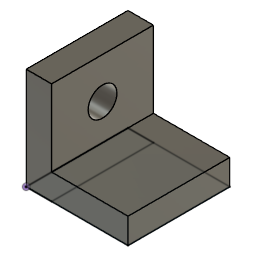
Final build (Autodesk Fusion 360 archive; units mm, degrees)
design "90 degree mount for coil housing"
part number: 2026-08-06-22-44-02-065
Autodesk Fusion 360 part; units mm, degrees
sketch "Sketch1" plane through (0, 0, 0) normal (0, 0, 1) x (1, 0, 0)
  line L0 (0, 0) -> (25.4, 0)
  line L1 (25.4, 0) -> (25.4, 25.4)
  line L2 (25.4, 25.4) -> (0, 25.4)
  line L3 (0, 25.4) -> (0, 0)
  line L4 (0, 25.4) -> (6.35, 25.4)
  line L5 (6.35, 25.4) -> (6.35, 0)
  line L6 (6.35, 0) -> (0, 0)
  line L7 (0, 0) -> (0, 25.4)
  dimension "d1" = 25.4
  dimension "d2" = 25.4
  dimension "d3" = 6.35
  constraint horizontal L0
  constraint vertical L1
  constraint horizontal L2
  constraint vertical L3
  constraint coincident L0.start L3.end
  constraint horizontal L4
  constraint vertical L5
  constraint horizontal L6
  constraint vertical L7
  constraint coincident L0 L5.end
  measures "d1" distance of L0.start L0.end
  measures "d2" distance of L0.start L2.end
  measures "d3" distance of L2.end L4.end
extrude "Extrude1" add sketch "Sketch1" along normal blind 6.35 contours L0 L1 L2 L5
extrude "Extrude2" add sketch "Sketch1" along normal blind 25.4 contours L0 L2 L3 L4 L5 L6 L7
sketch "Sketch2" plane through (6.35, 0, 0) normal (1, 0, 0) x (0, 1, 0)
  line L0 (0, 6.35) -> (25.4, 6.35)
  line L1 (25.4, 6.35) -> (25.4, 25.4)
  line L2 (25.4, 25.4) -> (0, 25.4)
  line L3 (0, 25.4) -> (0, 6.35)
  circle A0 centre (12.7, 15.24) radius 3.5921
extrude "Extrude3" cut sketch "Sketch2" against normal blind 38.1 contours A0

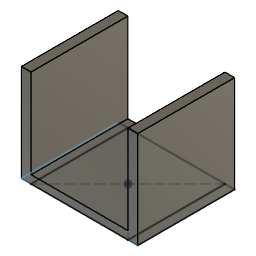
design "arm holder"
part number: 2026-08-05-14-50-43-195
Autodesk Fusion 360 part; units mm, degrees
sketch "Sketch1" plane through (0, 0, 0) normal (0, 0, 1) x (1, 0, 0)
  line L0 (38.1, 38.1) -> (-38.1, 38.1)
  line L1 (-38.1, 38.1) -> (-38.1, -38.1)
  line L2 (-38.1, -38.1) -> (38.1, -38.1)
  line L3 (38.1, -38.1) -> (38.1, 38.1)
  line L4 (38.1, 38.1) -> (-38.1, -38.1) construction
  line L5 (-38.1, 38.1) -> (38.1, -38.1) construction
  line L6 (-38.1, 38.1) -> (-45.72, 38.1)
  line L7 (-45.72, 38.1) -> (-45.72, -38.1)
  line L8 (-45.72, -38.1) -> (-38.1, -38.1)
  line L9 (-38.1, -38.1) -> (-38.1, 38.1)
  line L10 (38.1, 38.1) -> (45.72, 38.1)
  line L11 (45.72, 38.1) -> (45.72, -38.1)
  line L12 (45.72, -38.1) -> (38.1, -38.1)
  line L13 (38.1, -38.1) -> (38.1, 38.1)
  dimension "d1" = 76.2
  dimension "d2" = 76.2
  dimension "d3" = 7.62
  constraint horizontal L0
  constraint perpendicular L0 L1
  constraint parallel L0 L2
  constraint parallel L1 L3
  constraint coincident L4 origin
  constraint coincident L5 origin
  constraint horizontal L6
  constraint vertical L7
  constraint horizontal L8
  constraint vertical L9
  constraint horizontal L10
  constraint vertical L11
  constraint horizontal L12
  constraint vertical L13
  measures "d1" distance of L1.end L2.end
  measures "d2" distance of L0.end L1.end
  measures "d3" distance of L0.start L10.end
extrude "Extrude1" add sketch "Sketch1" along normal blind 6.35 contours L0 L1 L2 L3 L9 L13
sketch "Sketch2" plane through (0, 0, 0) normal (0, 0, 1) x (1, 0, 0)
extrude "Extrude2" add sketch "Sketch1" along normal blind 76.2 contours L3 L10 L11 L12 L13 | L1 L6 L7 L8 L9

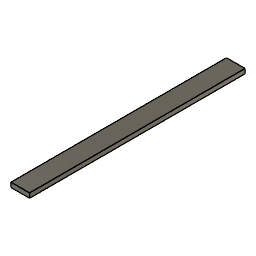
design "front and back side plates for coil housing"
part number: 2026-08-05-15-19-59-138
Autodesk Fusion 360 part; units mm, degrees
sketch "Sketch1" plane through (0, 0, 0) normal (0, 0, 1) x (1, 0, 0)
  line L0 (0, 0) -> (25.4, 0)
  line L1 (25.4, 0) -> (25.4, 293.37)
  line L2 (25.4, 293.37) -> (0, 293.37)
  line L3 (0, 293.37) -> (0, 0)
  dimension "d1" = 25.4
  dimension "d2" = 293.37
  constraint horizontal L0
  constraint vertical L1
  constraint horizontal L2
  constraint vertical L3
  constraint coincident L0.start L3.end
  measures "d1" distance of L0.start L0.end
  measures "d2" distance of L0.start L2.end
extrude "Extrude1" add sketch "Sketch1" along normal blind 6.35

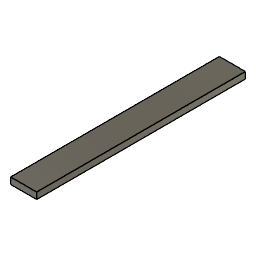
design "coil housing side plates"
part number: 2026-08-05-15-19-17-002
Autodesk Fusion 360 part; units mm, degrees
sketch "Sketch1" plane through (0, 0, 0) normal (0, 0, 1) x (1, 0, 0)
  line L0 (0, 0) -> (25.4, 0)
  line L1 (25.4, 0) -> (25.4, 203.2)
  line L2 (25.4, 203.2) -> (0, 203.2)
  line L3 (0, 203.2) -> (0, 0)
  dimension "d1" = 25.4
  dimension "d2" = 203.2
  constraint horizontal L0
  constraint vertical L1
  constraint horizontal L2
  constraint vertical L3
  constraint coincident L0.start L3.end
  measures "d1" distance of L0.start L0.end
  measures "d2" distance of L0.start L2.end
extrude "Extrude1" add sketch "Sketch1" along normal blind 6.35

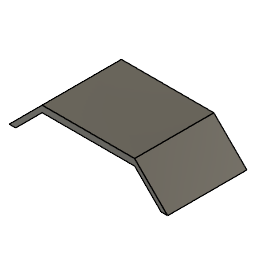
design "bottom bent plate"
part number: 2026-08-05-14-44-23-786
Autodesk Fusion 360 part; units mm, degrees
sketch "Sketch1" plane through (0, 0, 0) normal (0, 0, 1) x (1, 0, 0)
  line L0 (44.45, 38.1) -> (-44.45, 38.1)
  line L1 (-44.45, 38.1) -> (-44.45, -38.1)
  line L2 (-44.45, -38.1) -> (44.45, -38.1)
  line L3 (44.45, -38.1) -> (44.45, 38.1)
  line L4 (44.45, 38.1) -> (-44.45, -38.1) construction
  line L5 (-44.45, 38.1) -> (44.45, -38.1) construction
  dimension "d1" = 88.9
  dimension "d2" = 76.2
  constraint horizontal L0
  constraint perpendicular L0 L1
  constraint parallel L0 L2
  constraint parallel L1 L3
  constraint coincident L4 origin
  constraint coincident L5 origin
  measures "d1" distance of L1.end L2.end
  measures "d2" distance of L0.end L1.end
extrude "Extrude1" add sketch "Sketch1" along normal blind 6.35
sketch "Sketch2" plane through (0, 0, 0) normal (0, 1, 0) x (1, 0, 0)
  line L0 (44.45, -6.35) -> (76.2, 25.4)
  line L1 (44.45, 0) -> (69.85, 25.4)
  line L2 (69.85, 25.4) -> (76.2, 25.4)
  line L3 (0, -50.8) -> (0, 63.5)
  line L4 (-69.85, 25.4) -> (-76.2, 25.4)
  line L5 (-44.45, 0) -> (-69.85, 25.4)
  line L6 (-44.45, -6.35) -> (-76.2, 25.4)
  line L7 (-44.45, -6.35) -> (-44.45, 0)
  line L8 (44.45, -6.35) -> (44.45, 0)
  constraint parallel L0 L1
  constraint horizontal L2
  constraint vertical L3
  constraint symmetric L0.start L3 L6.start
  constraint symmetric L0.end L3 L4.end
  constraint symmetric L1.start L3 L5.start
  constraint symmetric L1.end L3 L4.start
  constraint vertical L7
extrude "Extrude2" add sketch "Sketch2" along normal blind 38.1 and the other way blind 38.1

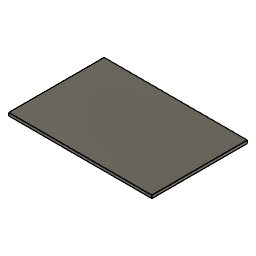
design "coil housing bottom and top plate"
part number: 2026-08-05-15-10-08-862
Autodesk Fusion 360 part; units mm, degrees
sketch "Sketch1" plane through (0, 0, 0) normal (0, 0, 1) x (1, 0, 0)
  line L0 (152.4, 101.6) -> (-152.4, 101.6)
  line L1 (-152.4, 101.6) -> (-152.4, -101.6)
  line L2 (-152.4, -101.6) -> (152.4, -101.6)
  line L3 (152.4, -101.6) -> (152.4, 101.6)
  line L4 (152.4, 101.6) -> (-152.4, -101.6) construction
  line L5 (-152.4, 101.6) -> (152.4, -101.6) construction
  dimension "d1" = 304.8
  dimension "d2" = 203.2
  constraint horizontal L0
  constraint perpendicular L0 L1
  constraint parallel L0 L2
  constraint parallel L1 L3
  constraint coincident L4 origin
  constraint coincident L5 origin
  measures "d1" distance of L1.end L2.end
  measures "d2" distance of L0.end L1.end
extrude "Extrude1" add sketch "Sketch1" along normal blind 6.35
